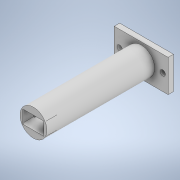
# Autodesk Inventor part: handle
Saved by Autodesk Inventor 2022 (Build 260153000, 153)
## iProperties
Created: 2022-01-31
Part Number: handle
Material: Generic
Document SubType Name: Modeling
Designer: Martijn
Density: 1 g/cm^3
Appearance: Default
Author: Martijn
Autodesk Inventor part; units mm, degrees
ref_plane "YZ Plane" through (0, 0, 0) normal (1, 0, 0) x (0, 1, 0)
ref_plane "XZ Plane" through (0, 0, 0) normal (0, 1, 0) x (-1, 0, 0)
ref_plane "XY Plane" through (0, 0, 0) normal (0, 0, 1) x (1, 0, 0)
sketch "Sketch1" plane through (0, 0, 0) normal (0, 0, 1) x (1, 0, 0)
  line L0 (0, 0) -> (50, 0)
  line L1 (50, 0) -> (50, 30)
  line L2 (50, 30) -> (0, 30)
  line L3 (0, 30) -> (0, 0)
  dimension "d0" = 30
  dimension "d1" = 50
  constraints: 8 end point, 2 parallel, 1 horizontal, 1 perpendicular
  measures "d0" distance of L2.end L0.start
  measures "d1" distance of L1.end L2.end
extrude "Extrusion1" add sketch "Sketch1" along normal blind 5
sketch "Sketch2" plane through (0, 0, 5) normal (0, 0, 1) x (1, 0, 0)
  circle A0 centre (25, 15) radius 12.5
  line L0 (0, 0) -> (50, 0) projected
  line L1 (0, 30) -> (0, 0) projected
  dimension "d5" = 25
  dimension "d6" = 15
  dimension "d7" = 25
  constraints: 1 centre point
  measures "d5" diameter of A0
  measures "d6" distance from line of L0 A0.centre
  measures "d7" distance from line of L1 A0.centre
extrude "Extrusion2" add sketch "Sketch2" along normal blind 100
sketch "Sketch3" plane through (25, 15, 105) normal (0, 0, 1) x (1, 0, 0)
  line L0 (-9.75, 6.1) -> (9.75, 6.1)
  line L1 (9.75, 6.1) -> (9.75, -6.1)
  line L2 (9.75, -6.1) -> (-9.75, -6.1)
  line L3 (-9.75, -6.1) -> (-9.75, 6.1)
  circle A0 centre (0, 0) radius 12.5 projected
  point P0 (-25, -15)
  dimension "d10" = 19.5
  dimension "d11" = 12.2
  dimension "d12" = 6.1
  dimension "d13" = 9.75
  constraints: 8 end point, 2 parallel, 1 coincident, 1 horizontal, 1 perpendicular
  measures "d10" distance of L0.start L0.end
  measures "d11" distance of L2.end L0.start
  measures "d12" vertical distance of L0.start point (0, 0)
  measures "d13" distance from line of point (0, 0) L3
extrude "Extrusion3" cut sketch "Sketch3" against normal blind 30 contours L0 L1 L2 L3
sketch "Sketch5" plane through (34.75, 8.9, 105) normal (-1, 0, 0) x (0, 0, 1)
  line L0 (0, 12.2) -> (-30, 12.2) projected
  line L1 (-1, 12.2) -> (-11, 12.2)
  line L2 (-11, 12.2) -> (-11, 0)
  line L3 (-11, 0) -> (-1, 0)
  line L4 (-1, 0) -> (-1, 12.2)
  line L5 (0, 0) -> (-30, 0) projected
  line L6 (0, 12.2) -> (0, 0) projected
  point P0 (-105, -8.9)
  dimension "d16" = 1
  dimension "d17" = 10
  constraints: 8 end point, 2 parallel, 2 point on line, 1 horizontal, 1 perpendicular
  measures "d16" distance between parallel lines of L6 L4
  measures "d17" distance between parallel lines of L4 L2
extrude "Extrusion4" cut sketch "Sketch5" against normal blind 1 contours L4 L3 L2 L0
sketch "Sketch6" plane through (15.25, 8.9, 105) normal (1, 0, 0) x (0, 0, -1)
  line L0 (0, 0) -> (30, 0) projected
  line L1 (0, 12.2) -> (30, 12.2) projected
  line L2 (1, 0) -> (11, 0)
  line L3 (11, 0) -> (11, 12.2)
  line L4 (11, 12.2) -> (1, 12.2)
  line L5 (1, 12.2) -> (1, 0)
  line L6 (0, 0) -> (0, 12.2) projected
  point P0 (105, -8.9)
  point P1 (1, 12.2)
  dimension "d20" = 1
  dimension "d21" = 10
  constraints: 8 end point, 2 parallel, 2 point on line, 1 horizontal, 1 perpendicular
  measures "d20" distance between parallel lines of L6 L5
  measures "d21" distance between parallel lines of L5 L3
extrude "Extrusion5" cut sketch "Sketch6" against normal blind 1 contours L5 L1 L3 L0
sketch "Sketch8" plane through (0, 0, 5) normal (0, 0, 1) x (1, 0, 0)
  circle A0 centre (5, 15) radius 2.5
  circle A1 centre (45, 15) radius 2.5
  line L0 (0, 0) -> (50, 0) projected
  line L1 (0, 30) -> (0, 0) projected
  line L2 (50, 0) -> (50, 30) projected
  line L3 (0, 0) -> (50, 0) projected
  point P0 (17, 0)
  point P1 (33, 0)
  dimension "d26" = 15
  dimension "d27" = 5
  dimension "d28" = 5
  dimension "d29" = 5
  dimension "d30" = 5
  dimension "d31" = 15
  constraints: 2 centre point
  measures "d26" distance from line of L0 A0.centre
  measures "d27" distance from line of L1 A0.centre
  measures "d28" diameter of A0
  measures "d29" diameter of A1
  measures "d30" distance from line of L2 A1.centre
  measures "d31" distance from line of L3 A1.centre
extrude "Extrusion7" cut sketch "Sketch8" against normal blind 10
sketch "Sketch9" plane through (25, 15, 75) normal (0, 0, 1) x (1, 0, 0)
  circle A0 centre (0, 0) radius 2.5
  line L0 (9.75, -6.1) -> (-9.75, -6.1) projected
  line L1 (9.75, 6.1) -> (9.75, -6.1) projected
  point P0 (-25, -15)
  dimension "d34" = 5
  dimension "d35" = 6.1
  dimension "d36" = 9.75
  constraints: 1 centre point
  measures "d34" diameter of A0
  measures "d35" distance from line of L0 A0.centre
  measures "d36" distance from line of L1 A0.centre
extrude "Extrusion8" cut sketch "Sketch9" against normal up to surface (75 mm away)
sketch "Sketch10" plane through (0, 0, 0) normal (-1, 0, 0) x (0, 0, 1)
  line L0 (5, 30) -> (5, 0) projected
  line L1 (5, 12.5) -> (10, 12.5)
  line L2 (10, 12.5) -> (10, 17.5)
  line L3 (10, 17.5) -> (5, 17.5)
  line L4 (5, 17.5) -> (5, 12.5)
  point P0 (0, 0)
  point P1 (5, 17.5)
  dimension "d39" = 5
  dimension "d40" = 12.5
  dimension "d41" = 5
  constraints: 8 end point, 2 parallel, 1 horizontal, 1 perpendicular, 1 point on line
  measures "d39" distance between parallel lines of L3 L1
  measures "d40" distance from line of L0.end L1
  measures "d41" distance between parallel lines of L0 L2
extrude "Extrusion9" cut sketch "Sketch10" against normal blind 25
equation "\"d13\" = 0.5 * d10"
body "Solid1"
